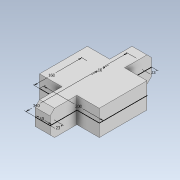
# Autodesk Inventor part: body_2
Saved by Autodesk Inventor 2020 (Build 240168000, 168)
## iProperties
Created: 2021-01-26
Part Number: body_2
Material: Generic
Document SubType Name: Modeling
Designer: DELL
Density: 1 g/cm^3
Appearance: Default
Author: DELL
Autodesk Inventor part; units mm, degrees
ref_plane "YZ Plane" through (0, 0, 0) normal (1, 0, 0) x (0, 1, 0)
ref_plane "XZ Plane" through (0, 0, 0) normal (0, 1, 0) x (-1, 0, 0)
ref_plane "XY Plane" through (0, 0, 0) normal (0, 0, 1) x (1, 0, 0)
sketch "Sketch1" plane through (0, 0, 0) normal (0, 1, 0) x (-1, 0, 0)
  line L0 (-100, -80) -> (-100, 80)
  line L1 (100, 80) -> (100, -80)
  line L2 (100, -80) -> (-100, 80) construction
  line L3 (-100, -80) -> (100, 80) construction
  line L4 (25, -170) -> (-25, -170)
  line L5 (-25, 170) -> (25, 170)
  line L6 (25, -170) -> (-25, 170) construction
  line L7 (-25, -170) -> (25, 170) construction
  line L8 (25, 170) -> (25, 80)
  line L9 (25, -80) -> (25, -170)
  line L10 (100, -80) -> (25, -80)
  line L11 (-25, -80) -> (-100, -80)
  line L12 (-25, -170) -> (-25, -80)
  line L13 (-25, 80) -> (-25, 170)
  line L14 (-100, 80) -> (-25, 80)
  line L15 (25, 80) -> (100, 80)
  line L16 (100, 0) -> (-100, 0) construction
  line L17 (0, -170) -> (0, 170) construction
  line L18 (15, -70) -> (90, -70)
  line L19 (90, -70) -> (90, 70)
  line L20 (90, 70) -> (15, 70)
  line L21 (15, 70) -> (15, 160)
  line L22 (15, 160) -> (-15, 160)
  line L23 (-15, 160) -> (-15, 70)
  line L24 (-15, 70) -> (-90, 70)
  line L25 (-90, 70) -> (-90, -70)
  line L26 (-90, -70) -> (-15, -70)
  line L27 (-15, -70) -> (-15, -160)
  line L28 (-15, -160) -> (15, -160)
  line L29 (15, -160) -> (15, -70)
  line L30 (15, -147) -> (-15, -147)
  line L31 (15, 147) -> (-15, 147)
  point P0 (0, 0)
  dimension "d0" = 50
  dimension "d1" = 200
  dimension "d2" = 340
  dimension "d3" = 160
  dimension "d9" = 10
  dimension "d10" = 23
  dimension "d11" = 23
  constraints: 64 end point, 20 parallel, 9 perpendicular, 8 midpoint, 4 horizontal, 4 point on line, 13 other
  measures "d0" distance of L5.start L5.end
  measures "d1" distance of L0.end L1.start
  measures "d2" distance of L5.end L4.start
  measures "d3" distance of L1.start L1.end
  measures "d9" distance between parallel lines of L10 L18
  measures "d10" distance between parallel lines of L5 L31
  measures "d11" distance between parallel lines of L4 L30
extrude "Extrusion1" add sketch "Sketch1" along normal mid plane 85 contours L0 L14 L13 L5 L8 L15 L1 L10 L9 L4 L12 L11 | L29 L30 L27 L26 L25 L24 L23 L31 L21 L20 L19 L18 | L29 L28 L27 L30 | L31 L23 L22 L21
chamfer "Chamfer1" distance 15 angle 45 4 edges at (0, 42.5, 170) (0, -42.5, 170) (0, 42.5, -170) (0, -42.5, -170)
extrude "Extrusion2" cut sketch "Sketch1" along normal mid plane 65 contours L29 L30 L27 L26 L25 L24 L23 L31 L21 L20 L19 L18
body "Solid1"
